Autodesk Inventor part; units mm, degrees
(part 2 of 2)
  line L823 (-45.1508, 120.65) -> (-47.9004, 115.8875)
  line L824 (-36.9019, 115.8875) -> (-39.6515, 120.65)
  line L825 (-39.6515, 111.125) -> (-36.9019, 115.8875)
  line L826 (-45.1508, 111.125) -> (-39.6515, 111.125)
  line L827 (-47.9004, 115.8875) -> (-45.1508, 111.125)
  line L828 (-39.6515, 107.95) -> (-45.1508, 107.95)
  line L829 (-45.1508, 107.95) -> (-47.9004, 103.1875)
  line L830 (-36.9019, 103.1875) -> (-39.6515, 107.95)
  line L831 (-39.6515, 98.425) -> (-36.9019, 103.1875)
  line L832 (-45.1508, 98.425) -> (-39.6515, 98.425)
  line L833 (-47.9004, 103.1875) -> (-45.1508, 98.425)
  line L834 (-39.6515, 95.25) -> (-45.1508, 95.25)
  line L835 (-45.1508, 95.25) -> (-47.9004, 90.4875)
  line L836 (-36.9019, 90.4875) -> (-39.6515, 95.25)
  line L837 (-39.6515, 85.725) -> (-36.9019, 90.4875)
  line L838 (-45.1508, 85.725) -> (-39.6515, 85.725)
  line L839 (-47.9004, 90.4875) -> (-45.1508, 85.725)
  line L840 (-39.6515, 82.55) -> (-45.1508, 82.55)
  line L841 (-45.1508, 82.55) -> (-47.9004, 77.7875)
  line L842 (-36.9019, 77.7875) -> (-39.6515, 82.55)
  line L843 (-39.6515, 73.025) -> (-36.9019, 77.7875)
  line L844 (-45.1508, 73.025) -> (-39.6515, 73.025)
  line L845 (-47.9004, 77.7875) -> (-45.1508, 73.025)
  line L846 (-39.6515, 69.85) -> (-45.1508, 69.85)
  line L847 (-45.1508, 69.85) -> (-47.9004, 65.0875)
  line L848 (-36.9019, 65.0875) -> (-39.6515, 69.85)
  line L849 (-39.6515, 60.325) -> (-36.9019, 65.0875)
  line L850 (-45.1508, 60.325) -> (-39.6515, 60.325)
  line L851 (-47.9004, 65.0875) -> (-45.1508, 60.325)
  line L852 (-39.6515, 57.15) -> (-45.1508, 57.15)
  line L853 (-45.1508, 57.15) -> (-47.9004, 52.3875)
  line L854 (-36.9019, 52.3875) -> (-39.6515, 57.15)
  line L855 (-39.6515, 47.625) -> (-36.9019, 52.3875)
  line L856 (-45.1508, 47.625) -> (-39.6515, 47.625)
  line L857 (-47.9004, 52.3875) -> (-45.1508, 47.625)
  line L858 (-39.6515, 44.45) -> (-45.1508, 44.45)
  line L859 (-45.1508, 44.45) -> (-47.9004, 39.6875)
  line L860 (-36.9019, 39.6875) -> (-39.6515, 44.45)
  line L861 (-39.6515, 34.925) -> (-36.9019, 39.6875)
  line L862 (-45.1508, 34.925) -> (-39.6515, 34.925)
  line L863 (-47.9004, 39.6875) -> (-45.1508, 34.925)
  line L864 (-39.6515, 31.75) -> (-45.1508, 31.75)
  line L865 (-45.1508, 31.75) -> (-47.9004, 26.9875)
  line L866 (-36.9019, 26.9875) -> (-39.6515, 31.75)
  line L867 (-39.6515, 22.225) -> (-36.9019, 26.9875)
  line L868 (-45.1508, 22.225) -> (-39.6515, 22.225)
  line L869 (-47.9004, 26.9875) -> (-45.1508, 22.225)
  line L870 (-39.6515, 19.05) -> (-45.1508, 19.05)
  line L871 (-45.1508, 19.05) -> (-47.9004, 14.2875)
  line L872 (-36.9019, 14.2875) -> (-39.6515, 19.05)
  line L873 (-39.6515, 9.525) -> (-36.9019, 14.2875)
  line L874 (-45.1508, 9.525) -> (-39.6515, 9.525)
  line L875 (-47.9004, 14.2875) -> (-45.1508, 9.525)
  line L876 (-24.4115, 120.65) -> (-29.9108, 120.65)
  line L877 (-29.9108, 120.65) -> (-32.6604, 115.8875)
  line L878 (-21.6619, 115.8875) -> (-24.4115, 120.65)
  line L879 (-24.4115, 111.125) -> (-21.6619, 115.8875)
  line L880 (-29.9108, 111.125) -> (-24.4115, 111.125)
  line L881 (-32.6604, 115.8875) -> (-29.9108, 111.125)
  line L882 (-24.4115, 107.95) -> (-29.9108, 107.95)
  line L883 (-29.9108, 107.95) -> (-32.6604, 103.1875)
  line L884 (-21.6619, 103.1875) -> (-24.4115, 107.95)
  line L885 (-24.4115, 98.425) -> (-21.6619, 103.1875)
  line L886 (-29.9108, 98.425) -> (-24.4115, 98.425)
  line L887 (-32.6604, 103.1875) -> (-29.9108, 98.425)
  line L888 (-24.4115, 95.25) -> (-29.9108, 95.25)
  line L889 (-29.9108, 95.25) -> (-32.6604, 90.4875)
  line L890 (-21.6619, 90.4875) -> (-24.4115, 95.25)
  line L891 (-24.4115, 85.725) -> (-21.6619, 90.4875)
  line L892 (-29.9108, 85.725) -> (-24.4115, 85.725)
  line L893 (-32.6604, 90.4875) -> (-29.9108, 85.725)
  line L894 (-24.4115, 82.55) -> (-29.9108, 82.55)
  line L895 (-29.9108, 82.55) -> (-32.6604, 77.7875)
  line L896 (-21.6619, 77.7875) -> (-24.4115, 82.55)
  line L897 (-24.4115, 73.025) -> (-21.6619, 77.7875)
  line L898 (-29.9108, 73.025) -> (-24.4115, 73.025)
  line L899 (-32.6604, 77.7875) -> (-29.9108, 73.025)
  line L900 (-24.4115, 69.85) -> (-29.9108, 69.85)
  line L901 (-29.9108, 69.85) -> (-32.6604, 65.0875)
  line L902 (-21.6619, 65.0875) -> (-24.4115, 69.85)
  line L903 (-24.4115, 60.325) -> (-21.6619, 65.0875)
  line L904 (-29.9108, 60.325) -> (-24.4115, 60.325)
  line L905 (-32.6604, 65.0875) -> (-29.9108, 60.325)
  line L906 (-24.4115, 57.15) -> (-29.9108, 57.15)
  line L907 (-29.9108, 57.15) -> (-32.6604, 52.3875)
  line L908 (-21.6619, 52.3875) -> (-24.4115, 57.15)
  line L909 (-24.4115, 47.625) -> (-21.6619, 52.3875)
  line L910 (-29.9108, 47.625) -> (-24.4115, 47.625)
  line L911 (-32.6604, 52.3875) -> (-29.9108, 47.625)
  line L912 (-24.4115, 44.45) -> (-29.9108, 44.45)
  line L913 (-29.9108, 44.45) -> (-32.6604, 39.6875)
  line L914 (-21.6619, 39.6875) -> (-24.4115, 44.45)
  line L915 (-24.4115, 34.925) -> (-21.6619, 39.6875)
  line L916 (-29.9108, 34.925) -> (-24.4115, 34.925)
  line L917 (-32.6604, 39.6875) -> (-29.9108, 34.925)
  line L918 (-24.4115, 31.75) -> (-29.9108, 31.75)
  line L919 (-29.9108, 31.75) -> (-32.6604, 26.9875)
  line L920 (-21.6619, 26.9875) -> (-24.4115, 31.75)
  line L921 (-24.4115, 22.225) -> (-21.6619, 26.9875)
  line L922 (-29.9108, 22.225) -> (-24.4115, 22.225)
  line L923 (-32.6604, 26.9875) -> (-29.9108, 22.225)
  line L924 (-24.4115, 19.05) -> (-29.9108, 19.05)
  line L925 (-29.9108, 19.05) -> (-32.6604, 14.2875)
  line L926 (-21.6619, 14.2875) -> (-24.4115, 19.05)
  line L927 (-24.4115, 9.525) -> (-21.6619, 14.2875)
  line L928 (-29.9108, 9.525) -> (-24.4115, 9.525)
  line L929 (-32.6604, 14.2875) -> (-29.9108, 9.525)
  line L930 (-9.1715, 120.65) -> (-14.6708, 120.65)
  line L931 (-14.6708, 120.65) -> (-17.4204, 115.8875)
  line L932 (-6.4219, 115.8875) -> (-9.1715, 120.65)
  line L933 (-9.1715, 111.125) -> (-6.4219, 115.8875)
  line L934 (-14.6708, 111.125) -> (-9.1715, 111.125)
  line L935 (-17.4204, 115.8875) -> (-14.6708, 111.125)
  line L936 (-9.1715, 107.95) -> (-14.6708, 107.95)
  line L937 (-14.6708, 107.95) -> (-17.4204, 103.1875)
  line L938 (-6.4219, 103.1875) -> (-9.1715, 107.95)
  line L939 (-9.1715, 98.425) -> (-6.4219, 103.1875)
  line L940 (-14.6708, 98.425) -> (-9.1715, 98.425)
  line L941 (-17.4204, 103.1875) -> (-14.6708, 98.425)
  line L942 (-9.1715, 95.25) -> (-14.6708, 95.25)
  line L943 (-14.6708, 95.25) -> (-17.4204, 90.4875)
  line L944 (-6.4219, 90.4875) -> (-9.1715, 95.25)
  line L945 (-9.1715, 85.725) -> (-6.4219, 90.4875)
  line L946 (-14.6708, 85.725) -> (-9.1715, 85.725)
  line L947 (-17.4204, 90.4875) -> (-14.6708, 85.725)
  line L948 (-9.1715, 82.55) -> (-14.6708, 82.55)
  line L949 (-14.6708, 82.55) -> (-17.4204, 77.7875)
  line L950 (-6.4219, 77.7875) -> (-9.1715, 82.55)
  line L951 (-9.1715, 73.025) -> (-6.4219, 77.7875)
  line L952 (-14.6708, 73.025) -> (-9.1715, 73.025)
  line L953 (-17.4204, 77.7875) -> (-14.6708, 73.025)
  line L954 (-9.1715, 69.85) -> (-14.6708, 69.85)
  line L955 (-14.6708, 69.85) -> (-17.4204, 65.0875)
  line L956 (-6.4219, 65.0875) -> (-9.1715, 69.85)
  line L957 (-9.1715, 60.325) -> (-6.4219, 65.0875)
  line L958 (-14.6708, 60.325) -> (-9.1715, 60.325)
  line L959 (-17.4204, 65.0875) -> (-14.6708, 60.325)
  line L960 (-9.1715, 57.15) -> (-14.6708, 57.15)
  line L961 (-14.6708, 57.15) -> (-17.4204, 52.3875)
  line L962 (-6.4219, 52.3875) -> (-9.1715, 57.15)
  line L963 (-9.1715, 47.625) -> (-6.4219, 52.3875)
  line L964 (-14.6708, 47.625) -> (-9.1715, 47.625)
  line L965 (-17.4204, 52.3875) -> (-14.6708, 47.625)
  line L966 (-9.1715, 44.45) -> (-14.6708, 44.45)
  line L967 (-14.6708, 44.45) -> (-17.4204, 39.6875)
  line L968 (-6.4219, 39.6875) -> (-9.1715, 44.45)
  line L969 (-9.1715, 34.925) -> (-6.4219, 39.6875)
  line L970 (-14.6708, 34.925) -> (-9.1715, 34.925)
  line L971 (-17.4204, 39.6875) -> (-14.6708, 34.925)
  line L972 (-9.1715, 31.75) -> (-14.6708, 31.75)
  line L973 (-14.6708, 31.75) -> (-17.4204, 26.9875)
  line L974 (-6.4219, 26.9875) -> (-9.1715, 31.75)
  line L975 (-9.1715, 22.225) -> (-6.4219, 26.9875)
  line L976 (-14.6708, 22.225) -> (-9.1715, 22.225)
  line L977 (-17.4204, 26.9875) -> (-14.6708, 22.225)
  line L978 (-9.1715, 19.05) -> (-14.6708, 19.05)
  line L979 (-14.6708, 19.05) -> (-17.4204, 14.2875)
  line L980 (-6.4219, 14.2875) -> (-9.1715, 19.05)
  line L981 (-9.1715, 9.525) -> (-6.4219, 14.2875)
  line L982 (-14.6708, 9.525) -> (-9.1715, 9.525)
  line L983 (-17.4204, 14.2875) -> (-14.6708, 9.525)
  point P0 (-142.875, -42.8625)
  point P1 (-133.8412, 115.8875)
  point P2 (-118.6012, 115.8875)
  point P3 (-103.3612, 115.8875)
  point P4 (-88.1212, 115.8875)
  point P5 (-72.8812, 115.8875)
  point P6 (-57.6412, 115.8875)
  point P7 (-42.4012, 115.8875)
  point P8 (-27.1612, 115.8875)
  point P9 (-11.9212, 115.8875)
  point P10 (-133.8412, 103.1875)
  point P11 (-118.6012, 103.1875)
  point P12 (-103.3612, 103.1875)
  point P13 (-88.1212, 103.1875)
  point P14 (-72.8812, 103.1875)
  point P15 (-57.6412, 103.1875)
  point P16 (-42.4012, 103.1875)
  point P17 (-27.1612, 103.1875)
  point P18 (-11.9212, 103.1875)
  point P19 (-133.8412, 90.4875)
  point P20 (-118.6012, 90.4875)
  point P21 (-103.3612, 90.4875)
  point P22 (-88.1212, 90.4875)
  point P23 (-72.8812, 90.4875)
  point P24 (-57.6412, 90.4875)
  point P25 (-42.4012, 90.4875)
  point P26 (-27.1612, 90.4875)
  point P27 (-11.9212, 90.4875)
  point P28 (-133.8412, 77.7875)
  point P29 (-118.6012, 77.7875)
  point P30 (-103.3612, 77.7875)
  point P31 (-88.1212, 77.7875)
  point P32 (-72.8812, 77.7875)
  point P33 (-57.6412, 77.7875)
  point P34 (-42.4012, 77.7875)
  point P35 (-27.1612, 77.7875)
  point P36 (-11.9212, 77.7875)
  point P37 (-133.8412, 65.0875)
  point P38 (-118.6012, 65.0875)
  point P39 (-103.3612, 65.0875)
  point P40 (-88.1212, 65.0875)
  point P41 (-72.8812, 65.0875)
  point P42 (-57.6412, 65.0875)
  point P43 (-42.4012, 65.0875)
  point P44 (-27.1612, 65.0875)
  point P45 (-11.9212, 65.0875)
  point P46 (-133.8412, 52.3875)
  point P47 (-118.6012, 52.3875)
  point P48 (-103.3612, 52.3875)
  point P49 (-88.1212, 52.3875)
  point P50 (-72.8812, 52.3875)
  point P51 (-57.6412, 52.3875)
  point P52 (-42.4012, 52.3875)
  point P53 (-27.1612, 52.3875)
  point P54 (-11.9212, 52.3875)
  point P55 (-133.8412, 39.6875)
  point P56 (-118.6012, 39.6875)
  point P57 (-103.3612, 39.6875)
  point P58 (-88.1212, 39.6875)
  point P59 (-72.8812, 39.6875)
  point P60 (-57.6412, 39.6875)
  point P61 (-42.4012, 39.6875)
  point P62 (-27.1612, 39.6875)
  point P63 (-11.9212, 39.6875)
  point P64 (-133.8412, 26.9875)
  point P65 (-118.6012, 26.9875)
  point P66 (-103.3612, 26.9875)
  point P67 (-88.1212, 26.9875)
  point P68 (-72.8812, 26.9875)
  point P69 (-57.6412, 26.9875)
  point P70 (-42.4012, 26.9875)
  point P71 (-27.1612, 26.9875)
  point P72 (-11.9212, 26.9875)
  point P73 (-133.8412, 14.2875)
  point P74 (-118.6012, 14.2875)
  point P75 (-103.3612, 14.2875)
  point P76 (-88.1212, 14.2875)
  point P77 (-72.8812, 14.2875)
  point P78 (-57.6412, 14.2875)
  point P79 (-42.4012, 14.2875)
  point P80 (-27.1612, 14.2875)
  point P81 (-11.9212, 14.2875)
  point P82 (-17.4204, 119.0625)
  point P83 (-21.6619, 119.0625)
  point P84 (-32.6604, 119.0625)
  point P85 (-36.9019, 119.0625)
  point P86 (-47.9004, 119.0625)
  point P87 (-52.1419, 119.0625)
  point P88 (-63.1404, 119.0625)
  point P89 (-67.3819, 119.0625)
  point P90 (-78.3804, 119.0625)
  point P91 (-82.6219, 119.0625)
  point P92 (-124.1004, 119.0625)
  point P93 (-128.3419, 119.0625)
  point P94 (-108.8604, 119.0625)
  point P95 (-113.1019, 119.0625)
  point P96 (-93.6204, 119.0625)
  point P97 (-97.8619, 119.0625)
  point P98 (-7.9375, 11.6624)
  point P99 (-7.9375, 16.9126)
  point P100 (-7.9375, 37.0624)
  point P101 (-7.9375, 42.3126)
  point P102 (-7.9375, 49.7624)
  point P103 (-7.9375, 55.0126)
  point P104 (-7.9375, 62.4624)
  point P105 (-7.9375, 67.7126)
  point P106 (-7.9375, 75.1624)
  point P107 (-7.9375, 80.4126)
  point P108 (-7.9375, 87.8624)
  point P109 (-7.9375, 93.1126)
  point P110 (-7.9375, 100.5624)
  point P111 (-7.9375, 105.8126)
  point P112 (-69.215, 119.0625)
  point P113 (-76.5473, 119.0625)
  point P114 (-99.695, 119.0625)
  point P115 (-107.0273, 119.0625)
  point P116 (-138.1125, 92.6143)
  point P117 (-138.1125, 88.3607)
  point P118 (-138.1125, 79.9143)
  point P119 (-138.1125, 75.6607)
  point P120 (-138.1125, 67.2143)
  point P121 (-138.1125, 62.9607)
  point P122 (-138.1125, 54.5143)
  point P123 (-138.1125, 50.2607)
  dimension "d20" = 15.24
  dimension "d23" = 12.7
  dimension "d28" = 12.7
  dimension "d31" = 15.24
  constraints: 1964 end point, 432 horizontal alignment, 292 parallel, 144 collinear, 4 horizontal, 2 perpendicular, 1 point on line, 1 vertical, 121 other
  measures "d20" distance of point (-133.841, 115.888) point (-118.601, 115.888)
  measures "d23" distance of point (-133.841, 115.888) point (-133.841, 103.188)
  measures "d28" distance of L499.end L504.start
  measures "d31" distance of L499.end L552.start
extrude "Extrusion5" cut sketch "Sketch5" against normal blind 49.53 contours L496 L13 L12 L67 L66 L121 L120 L175 L174 L229 L228 L283 L282 L337 L336 L391 L390 L445 L444 L494 L436 L435 L382 L381 L328 L327 L274 L273 L220 L219 L166 L165 L112 L111 L58 L57 L4 L3 | L499 L498 L503 L502 L495 L501 L496 | L496 L501 L500 L499 | L553 L552 L554 L496 | L496 L554 L555 L556 L557 L553 | L495 L502 L501 | L10 L9 L496 L19 L18 L73 L72 L127 L126 L181 L180 L235 L234 L289 L288 L343 L342 L397 L396 L451 L450 L494 L442 L441 L388 L387 L334 L333 L280 L279 L226 L225 L172 L171 L118 L117 L64 L63 | L505 L504 L506 L507 L508 L509 L495 | L495 L509 L505 | L496 L608 L609 L610 L611 L607 | L511 L510 L512 L513 L514 L515 L495 | L16 L15 L496 L25 L24 L79 L78 L133 L132 L187 L186 L241 L240 L295 L294 L349 L348 L403 L402 L457 L456 L494 L448 L447 L394 L393 L340 L339 L286 L285 L232 L231 L178 L177 L124 L123 L70 L69 | L517 L516 L518 L519 L520 L521 L495 | L661 L660 L662 L496 | L496 L662 L663 L664 L665 L661 | L523 L522 L524 L525 L526 L527 L495 | L22 L21 L496 L31 L30 L85 L84 L139 L138 L193 L192 L247 L246 L301 L300 L355 L354 L409 L408 L463 L462 L494 L454 L453 L400 L399 L346 L345 L292 L291 L238 L237 L184 L183 L130 L129 L76 L75 | L529 L528 L530 L531 L532 L533 L495 | L496 L716 L717 L718 L719 L715 | L535 L534 L536 L537 L538 L539 L495 | L495 L539 L535 | L28 L27 L496 L37 L36 L91 L90 L145 L144 L199 L198 L253 L252 L307 L306 L361 L360 L415 L414 L469 L468 L494 L460 L459 L406 L405 L352 L351 L298 L297 L244 L243 L190 L189 L136 L135 L82 L81 | L541 L540 L542 L543 L544 L545 L495 | L495 L545 L541 | L769 L768 L770 L496 | L496 L770 L771 L772 L773 L769 | L547 L546 L548 L549 L550 L551 L495 | L495 L551 L547 | L34 L33 L496 L43 L42 L97 L96 L151 L150 L205 L204 L259 L258 L313 L312 L367 L366 L421 L420 L475 L474 L494 L466 L465 L412 L411 L358 L357 L304 L303 L250 L249 L196 L195 L142 L141 L88 L87 | L823 L822 L824 L496 | L496 L824 L825 L826 L827 L823 | L40 L39 L496 L49 L48 L103 L102 L157 L156 L211 L210 L265 L264 L319 L318 L373 L372 L427 L426 L481 L480 L494 L472 L471 L418 L417 L364 L363 L310 L309 L256 L255 L202 L201 L148 L147 L94 L93 | L877 L876 L878 L496 | L496 L878 L879 L880 L881 L877 | L46 L45 L496 L55 L54 L109 L108 L163 L162 L217 L216 L271 L270 L325 L324 L379 L378 L433 L432 L487 L486 L494 L478 L477 L424 L423 L370 L369 L316 L315 L262 L261 L208 L207 L154 L153 L100 L99 | L931 L930 L932 L496 | L496 L932 L497 L933 L934 L935 L931 | L932 L933 L497 | L497 L939 L940 L941 L937 L936 L938 | L981 L982 L983 L979 L978 L980 L497 | L497 L945 L946 L947 L943 L942 L944 | L975 L976 L977 L973 L972 L974 L497 | L497 L974 L975 | L497 L951 L952 L953 L949 L948 L950 | L969 L970 L971 L967 L966 L968 L497 | L497 L957 L958 L959 L955 L954 L956 | L963 L964 L965 L961 L960 L962 L497 | L560 L561 L562 L563 L559 L558 | L566 L567 L568 L569 L565 L564 | L572 L573 L574 L575 L571 L570 | L578 L579 L580 L581 L577 L576 | L584 L585 L586 L587 L583 L582 | L590 L591 L592 L593 L589 L588 | L596 L597 L598 L599 L595 L594 | L602 L603 L604 L605 L601 L600 | L614 L615 L616 L617 L613 L612 | L620 L621 L622 L623 L619 L618 | L626 L627 L628 L629 L625 L624 | L632 L633 L634 L635 L631 L630 | L638 L639 L640 L641 L637 L636 | L644 L645 L646 L647 L643 L642 | L650 L651 L652 L653 L649 L648 | L656 L657 L658 L659 L655 L654 | L668 L669 L670 L671 L667 L666 | L674 L675 L676 L677 L673 L672 | L680 L681 L682 L683 L679 L678 | L686 L687 L688 L689 L685 L684 | L692 L693 L694 L695 L691 L690 | L698 L699 L700 L701 L697 L696 | L704 L705 L706 L707 L703 L702 | L710 L711 L712 L713 L709 L708 | L722 L723 L724 L725 L721 L720 | L728 L729 L730 L731 L727 L726 | L734 L735 L736 L737 L733 L732 | L740 L741 L742 L743 L739 L738 | L746 L747 L748 L749 L745 L744 | L752 L753 L754 L755 L751 L750 | L758 L759 L760 L761 L757 L756 | L764 L765 L766 L767 L763 L762 | L776 L777 L778 L779 L775 L774 | L782 L783 L784 L785 L781 L780 | L788 L789 L790 L791 L787 L786 | L794 L795 L796 L797 L793 L792 | L800 L801 L802 L803 L799 L798 | L806 L807 L808 L809 L805 L804 | L812 L813 L814 L815 L811 L810 | L818 L819 L820 L821 L817 L816 | L830 L831 L832 L833 L829 L828 | L836 L837 L838 L839 L835 L834 | L842 L843 L844 L845 L841 L840 | L848 L849 L850 L851 L847 L846 | L854 L855 L856 L857 L853 L852 | L860 L861 L862 L863 L859 L858 | L866 L867 L868 L869 L865 L864 | L872 L873 L874 L875 L871 L870 | L884 L885 L886 L887 L883 L882 | L890 L891 L892 L893 L889 L888 | L896 L897 L898 L899 L895 L894 | L902 L903 L904 L905 L901 L900 | L908 L909 L910 L911 L907 L906 | L914 L915 L916 L917 L913 L912 | L920 L921 L922 L923 L919 L918 | L926 L927 L928 L929 L925 L924
body "Solid1"
